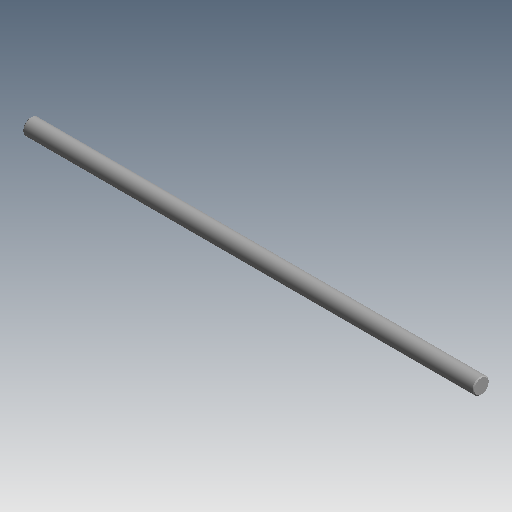
# Autodesk Inventor part: SSFR10-280_s
Saved by Autodesk Inventor 2020.1 (Build 241239000, 239)
## iProperties
Part Number: SSFR10-280_s
Material: 一般
Catalog Web Link: www.cadenas.de
Description: NSFMR, SFMR, PSFMR, SSFMR, NSFHR, SFHR, PSFHR, SSFHR, NSFR, SFR, PSFR, SSFR, HFR, PHFR_shaft-Rotary Shafts - Straight -
Vendor: MISUMI
Document SubType Name: Modeling
Designer: partserver
Manufacturer: MISUMI
Mass: 21.9836 g
Surface Area: 89.3449 cm^2
Volume: 21.9836 cm^3
Density: 1 g/cm^3
Appearance: PSOLRGB-192-192-192
Category: PARTsolutions
Company: MISUMI
PSOL_IDENT_0: {$CADENAS_DATA\23d-libs\misumi\metric\11_rotary_shafts\11_components\psfr\psfr.prj},460 {VTYP=3D},{N
PSOL_IDENT_1: B=SSFR10-280_s},{LINA=SSFR10-280},{NN=NSFMR, SFMR, PSFMR, SSFMR, NSFHR, SFHR, PSFHR, SSFHR, NSFR, SF
PSOL_IDENT_2: R, PSFR, SSFR, HFR, PHFR_shaft},{DATE=19.04.2020 19:01:32},{GEOMDATE=17.04.2020 07:28:52},{VERSION=}
PSOL_IDENT_3: ,{LINEID=30},{WBVAR=TS,MAT,ST,ALT1,L,ALT2,KC,A,WKC,C,K,E,KZ,Z,ALT3,FC,GALT3,WFC,J,WALT3,V,ALT4,SFC,S
PSOL_IDENT_4: G,AG,ALT10,KWC,ALT11,WC,ALT6,TA,TB,ALT5,UC,ALT7,SC,ALT32,CD},{WBNUMERIC=L,KC,A,WKC,C,K,E,KZ,Z,FC,GAL
PSOL_IDENT_5: T3,WFC,J,WALT3,V,SFC,SG,AG,KWC,WC,TA,TB,UC,SC}  {NB=SSFR10-280_s},{LINA=SSFR10-280},{KT=DUMMY},{PN=S
PSOL_IDENT_6: SFR10-280},{TYPE=SSFR},{TS=},{TSALG='M','h9 (Cold-drawn)','H','h7 (Ground)','','g6 (Ground)'},{MAT=S
PSOL_IDENT_7: US304},{MATALG= 'S45C','S45C Equivalent', 'SUS304','SUS304' },{ST=-},{STALG= '-','-' },{D=10.0},{ALT
PSOL_IDENT_8: 1=},{L=280.0},{LALG=[15:800/0.1]},{LMIN=15},{LMAX=800},{ALT2=},{ALT2ALG= '', 'w/o Key Grooves','KC','
PSOL_IDENT_9: with KC (Key Groove)','WKC','with WKC (Two Key Grooves)','KCWKC','with KC + WKC (Three Key Grooves)'
PSOL_IDENT_10: ,'KZ','with KC + WKC + KZ (Four Key Grooves)' },{ALT2PN=},{KC=0.0},{KCALG=[0]},{KCMIN=0},{KCMAX=0},{
PSOL_IDENT_11: A=0.0},{AALG=[0]},{AMIN=3},{AMAX=0},{WKC=0.0},{WKCALG=[0]},{WKCMIN=0},{WKCMAX=0},{C=0.0},{CALG=[0]},
PSOL_IDENT_12: {CMIN=3},{CMAX=0},{K=0.0},{KALG=[0]},{KMIN=0},{KMAX=275},{E=0.0},{EALG=[0]},{EMIN=3},{EMAX=100},{KZ=
PSOL_IDENT_13: 0.0},{KZALG=[0]},{KZMIN=282},{KZMAX=277},{Z=0.0},{ZALG=[0]},{ZMIN=3},{ZMAX=100},{CIFKC=1},{CIFWKC=1}
PSOL_IDENT_14: ,{CIFK=1},{CIFKZ=2},{PCUT3D=0.000},{QCUT3D=0},{BB=3},{BBALT2=3},{TT=1.8},{TTALT2=1.8},{ALT3=},{ALT3A
PSOL_IDENT_15: LG= '', 'w/o Set Screw Flat','FC','with FC (Adds a Set Screw Flat)','WFC','with WFC (Adds Two Set Sc
PSOL_IDENT_16: rew Flats)','FCWFC','with FC + WFC (Adds Three Set Screw Flats)' },{ALT3PN=},{FC=0},{FCALG=[0]},{FCM
PSOL_IDENT_17: IN=0},{FCMAX=279},{GALT3=0},{GALT3ALG=[0]},{GALT3MIN=1},{GALT3MAX=70},{GALT3MAX2=70},{GALT3MAX3=70},
PSOL_IDENT_18: {WFC=0},{WFCALG=[0]},{WFCMIN=0},{WFCMIN2=2},{WFCMAX=276},{WFCMAX2=-3},{WFCMAX3=-4},{J=0},{JALG=[0]},
PSOL_IDENT_19: {JMIN=1},{JMAX=70},{JMAX2=-2},{JMAX3=-5},{WALT3=0},{WALT3ALG=[0]},{WALT3MIN=0},{WALT3MIN2=282},{WALT
PSOL_IDENT_20: 3MAX=277},{WALT3MAX2=277},{WALT3MAX3=277},{V=0},{VALG=[0]},{VMIN=1},{VMAX=70},{VMAX2=70},{VMAX3=50},
PSOL_IDENT_21: {CIFFC=0},{ALT4=},{ALT4ALG= '', 'w/o SFC (2 Set Screw Flats (Angle Specified))', 'SFC'  , 'with SFC
PSOL_IDENT_22: (2 Set Screw Flats (Angle Specified))'},{ALT4PN=},{SFC=0},{SFCALG=[0]},{SFCMIN=0},{SFCMAX=279},{SG=0
PSOL_IDENT_23: },{SGALG=[0]},{SGMIN=1},{SGMAX=70},{AG=0},{AGALG=[0]},{H=0.0},{CIFSFC=0},{ALT10=},{ALT10ALG= '', 'w/
PSOL_IDENT_24: o KWC (2 Set Screw Flats at both ends)', 'KWC', 'with KWC (2 Set Screw Flats at both ends)' },{ALT10
PSOL_IDENT_25: PN=},{KWC=0},{KWCALG=[0]},{KWCMIN=1},{KWCMAX=139},{WALT10=8},{ALT11=},{ALT11ALG= '','Not applicable'
PSOL_IDENT_26: },{ALT11PN=},{WC=0.0},{WCALG=[0]},{ALT6=},{ALT6ALG= '','w/o Retaining Ring Groove','TA','with TA (R
PSOL_IDENT_27: etaining Ring Groove)','TB','with TB (Retaining Ring Groove)','TATB','with TA + TB (Two Retaining Ri
PSOL_IDENT_28: ng Grooves)' },{ALT6PN=},{TA=0.0},{TAALG=[0]},{TAMIN=2},{TAMAX=0},{TB=0.0},{TBALG=[0]},{TBMIN=2},{TB
PSOL_IDENT_29: MAX=0},{DDALT6=0.0},{MM=0.00},{ALT5=},{ALT5ALG= '', 'w/o UC (Slit Cam Groove)', 'UC', 'with UC (Slit
PSOL_IDENT_30: Cam Groove)'},{ALT5PN=},{UC=0},{UCALG=[0]},{UCMIN=1},{UCMAX=274},{DDALT5=0},{LL1=0},{ALT7=},{ALT7AL
PSOL_IDENT_31: G= '', 'w/o SC (Wrench Flats)', 'SC', 'with SC (Wrench Flats)'},{ALT7PN=},{SC=0},{SCALG=[0]},{SCMIN=
PSOL_IDENT_32: 0},{SCMAX=272},{WALT7=0},{LL2=0},{LL2ALG=8},{CIFSC=0},{ALT32=},{ALT32ALG=  '','w/o CD (Changes Part
PSOL_IDENT_33: D Chamfering)','-CD', 'with CD (Changes Part D Chamfering)' },{ALT32PN=},{CD=},{CDALG= '','N/A' },{C
PSOL_IDENT_34: D3D=0.5},{CIF32=0},{CIF320=0},{CIFTA=0},{CIFTB=0},{ERRORPN=},{ERRORALT23=OK},{ERRORALT24=OK},{ERRORA
PSOL_IDENT_35: LT25=OK},{ERRORALT26=OK},{ERRORALT27=OK},{ERRORALT210=OK},{ERRORALT34=OK},{ERRORALT35=OK},{ERRORALT3
PSOL_IDENT_36: 6=OK},{ERRORALT37=OK},{ERRORALT310=OK},{ERRORALT45=OK},{ERRORALT46=OK},{ERRORALT47=OK},{ERRORALT410=
PSOL_IDENT_37: OK},{ERRORALT56=OK},{ERRORALT57=OK},{ERRORALT510=OK},{ERRORALT610=OK},{ERRORALT75=OK},{ERRORALT76=OK
PSOL_IDENT_38: },{ERRORALT710=OK}
NB: SSFR10-280_s
NN: NSFMR, SFMR, PSFMR, SSFMR, NSFHR, SFHR, PSFHR, SSFHR, NSFR, SFR, PSFR, SSFR, HFR, PHFR_shaft
NT: Rotary Shafts - Straight -
NBSYN: $PN._s
LINA: SSFR10-280
CATALOG: Misumi
PN: SSFR10-280
TS: g6 (Ground)
MAT: SUS304
ST: -
D: 10
ALT1: w/o LKC (Changes L Tolerance)
L: 280
ALT2: w/o Key Grooves
KC: 0
A: 0
WKC: 0
C: 0
K: 0
E: 0
KZ: 0
Z: 0
ALT3: w/o Set Screw Flat
FC: 0
GALT3: 0
WFC: 0
J: 0
WALT3: 0
V: 0
ALT4: w/o SFC (2 Set Screw Flats (Angle Specified))
SFC: 0
SG: 0
AG: 0
H: 0
ALT10: w/o KWC (2 Set Screw Flats at both ends)
KWC: 0
ALT11: Not applicable
WC: 0
ALT6: w/o Retaining Ring Groove
TA: 0
TB: 0
DDALT6: 0
MM: 0
ALT5: w/o UC (Slit Cam Groove)
UC: 0
DDALT5: 0
LL1: 0
ALT7: w/o SC (Wrench Flats)
SC: 0
WALT7: 0
LL2: 0
ALT32: w/o CD (Changes Part D Chamfering)
CD: N/A
SUPPLIER: MISUMI
ARTICLENO: SSFR10-280_s
BOMINFO: SSFR10-280
CREATOR: CADENAS GmbH
Title: SSFR10-280
Author: Cadenas PARTsolutions
Comments: Rotary Shafts - Straight -
Autodesk Inventor part; units mm, degrees
sketch "Sketch_1" plane through (0, 0, 0) normal (0, 0, 1) x (1, 0, 0)
  line L0 (280, 0) -> (0, 0)
  line L1 (0, 0) -> (0, 4.5)
  line L2 (0, 4.5) -> (0.5, 5)
  line L3 (0.5, 5) -> (279.5, 5)
  line L4 (279.5, 5) -> (280, 4.5)
  line L5 (280, 4.5) -> (280, 0)
  line L6 (280, 0) -> (0, 0)
  constraints: 14 end point
revolve "Revolution1" add sketch "Sketch_1" angle 360 about axis through (280, 0, 0) along (1, 0, 0)
ref_plane "COMBINATION_MODULE_XY" through (0, 0, 0) normal (1, 0, 0) x (0, 0, -1)
ref_plane "COMBINATION_MODULE_YZ" through (0, 0, 0) normal (0, 0, -1) x (0, 1, 0)
ref_plane "COMBINATION_MODULE_ZX" through (0, 0, 0) normal (0, 1, 0) x (1, 0, 0)
body "Solid1"
